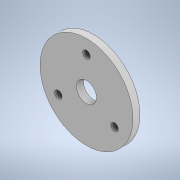
# Autodesk Inventor part: bearing_holder2
Saved by Autodesk Inventor 2020.3 (Build 243373000, 373)
## iProperties
Created: 2020-11-01
Part Number: bearing_holder2
Material: Generic
Document SubType Name: Modeling
Designer: Martijn
Density: 1 g/cm^3
Appearance: Default
Author: Martijn
Autodesk Inventor part; units mm, degrees
ref_plane "YZ Plane" through (0, 0, 0) normal (1, 0, 0) x (0, 1, 0)
ref_plane "XZ Plane" through (0, 0, 0) normal (0, 1, 0) x (-1, 0, 0)
ref_plane "XY Plane" through (0, 0, 0) normal (0, 0, 1) x (1, 0, 0)
sketch "Sketch1" plane through (0, 0, 0) normal (0, 0, 1) x (1, 0, 0)
  circle A0 centre (0, 0) radius 20
  circle A1 centre (0, 0) radius 4.3
  dimension "d0" = 40
  dimension "d2" = 8.6
  constraints: 2 centre point, 2 coincident
  measures "d0" diameter of A0
  measures "d2" diameter of A1
extrude "Extrusion1" add sketch "Sketch1" along normal blind 3
sketch "Sketch2" plane through (0, 0, 3) normal (0, 0, 1) x (1, 0, 0)
  circle A0 centre (0, 14) radius 1.6
  line L0 (0, -28) -> (0, 28) projected
  point P0 (0, 0)
  dimension "d5" = 14
  dimension "d6" = 3.2
  constraints: 1 centre point, 1 point on line
  measures "d5" distance of point (0, 0) A0.centre
  measures "d6" diameter of A0
extrude "Extrusion2" cut sketch "Sketch2" against normal blind 10
pattern_circular "Circular Pattern1" count 3 over 360 about axis through (0, 0, 0) along (0, 0, 1) of "Extrusion2"
body "Solid1"
